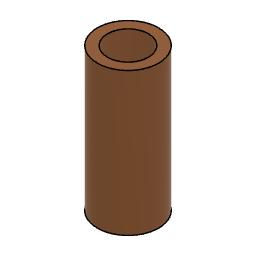
electrode puck v2 vespel spacer v2 (Autodesk Fusion 360 design; units mm, degrees)
Autodesk Fusion 360 part; units mm, degrees
cylinder "CylinderPrimitive1" add diameter 3 height 7 placed x (1, 0, 0) y (0, 0, -1) z (0, 1, 0) at (0, 0, 0)
cylinder "CylinderPrimitive2" cut diameter 2 height 7.5 placed x (1, 0, 0) y (0, 0, -1) z (0, 1, 0) at (0, 0, 0)
